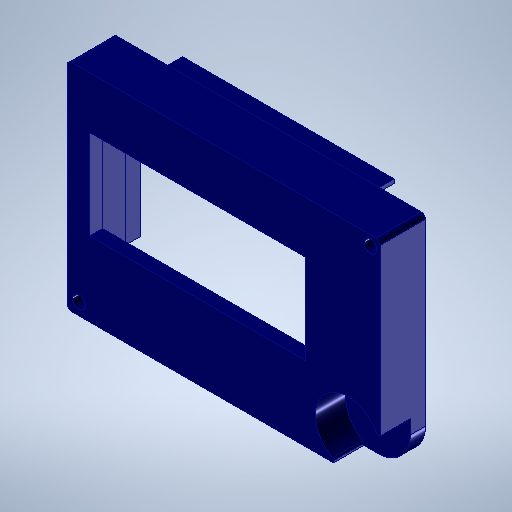
# Autodesk Inventor part: Krabička_horni
Saved by Autodesk Inventor 2025.2 (Build 292293000, 293)
## iProperties
Created: 2025-03-25
Part Number: Krabička_horni
Material: Všeobecné
Document SubType Name: Modeling
Designer: jakub
Density: 1 g/cm^3
Appearance: Modrá – nástěnná malba – lesklá
Author: jakub
## iProperties of the stored document Krabička_horni_3D tisk.ipt
Created: 2025-03-26
Part Number: Krabička_horni_3D tisk
Material: Všeobecné
Document SubType Name: Modeling
Designer: jakub
Density: 1 g/cm^3
Appearance: Výchozí
Author: jakub
Autodesk Inventor part; units mm, degrees
ref_plane "YZ Plane" through (0, 0, 0) normal (1, 0, 0) x (0, 1, 0)
ref_plane "XZ Plane" through (0, 0, 0) normal (0, 1, 0) x (-1, 0, 0)
ref_plane "XY Plane" through (0, 0, 0) normal (0, 0, 1) x (1, 0, 0)
sketch "Náčrt1" plane through (0, 0, 0) normal (0, 0, 1) x (1, 0, 0)
  line L0 (0, 71.1184) -> (0, -73.8108) projected
  line L1 (-102.6184, 0) -> (105.3108, 0) projected
  line L2 (-72.5, 50) -> (72.5, 50)
  line L3 (72.5, 50) -> (72.5, -35)
  line L4 (57.5, -50) -> (-72.5, -50)
  line L5 (-72.5, -50) -> (-72.5, 50)
  arc A0 (57.5, -50) -> (72.5, -35) centre (57.5, -35) ccw
  point P0 (0, 0)
  dimension "d2" = 30
  dimension "d37" = 145
  dimension "d38" = 100
  constraints: 8 end point, 2 parallel, 2 point on circle, 2 tangent, 1 centre point, 1 horizontal, 1 perpendicular, 2 other
  measures "d2" diameter of A0
  measures "d37" distance between parallel lines of L3 L5
  measures "d38" distance between parallel lines of L2 L4
extrude "Vysunutí1" add sketch "Náčrt1" along normal blind 21
sketch "Náčrt2" plane through (0, 0, 21) normal (0, 0, 1) x (1, 0, 0)
  line L0 (-72.5, -50) -> (57.5, -50) projected
  arc A0 (57.5, -50) -> (72.5, -35) centre (57.5, -35) ccw projected
  line L1 (72.5, -35) -> (72.5, 50) projected
  line L2 (72.5, 50) -> (-72.5, 50) projected
  line L3 (-72.5, 50) -> (-72.5, -50) projected
  circle A1 centre (57.5, -35) radius 15
  line L4 (72.5, -27.3264) -> (72.5, -35)
  line L5 (64.2851, -50) -> (57.5, -50)
  line L6 (72.5, -35) -> (72.5, 50) projected
  line L7 (72.5, -35) -> (72.5, -35)
  line L8 (72.5, -28.4617) -> (71, -28.4617)
  line L9 (50.9617, -48.5) -> (50.9617, -50)
  point P0 (0, 0)
  point P1 (49.2851, -47.5505)
  point P2 (70.3886, -27.3264)
  point P3 (50.9617, -50)
  dimension "d11" = 1.5
  dimension "d12" = 1.5
  constraints: 10 end point, 5 point on circle, 5 point on line, 4 perpendicular, 4 tangent, 1 centre point, 1 coincident, 1 collinear, 1 concentric
  measures "d11" distance of L8.start L8.end
  measures "d12" distance of L9.start L9.end
extrude "Vysunutí2" cut sketch "Náčrt2" against normal blind 14 contours L9 A1 L0 | A1 A0 | A1 L8 L1
sketch "Náčrt3" plane through (0, 0, 7) normal (0, 0, 1) x (1, 0, 0)
  arc A0 (57.5, -50) -> (72.5, -35) centre (57.5, -35) ccw projected
  circle A1 centre (57.5, -35) radius 4.25
  line L0 (72.5, -28.4617) -> (72.5, -35) projected
  line L1 (57.5, -50) -> (50.9617, -50) projected
  line L2 (71, -28.4617) -> (72.5, -28.4617) projected
  arc A2 (71, -28.4617) -> (50.9617, -48.5) centre (57.5, -35) ccw projected
  line L3 (50.9617, -50) -> (50.9617, -48.5) projected
  point P0 (0, 0)
  dimension "d7" = 8.5
  constraints: 1 centre point, 1 coincident
  measures "d7" diameter of A1
extrude "Vysunutí3" cut sketch "Náčrt3" against normal blind 12 contours A1
fillet "Zaoblení1" radius 2 3 edges at (72.5, 50, 10.5) (-72.5, 50, 10.5) (-72.5, -50, 10.5)
fillet "Zaoblení2" radius 1 2 edges at (71, -28.4617, 14) (50.9617, -48.5, 14)
sketch "Náčrt4" plane through (0, 0, 21) normal (0, 0, 1) x (1, 0, 0)
  arc A0 (50.9617, -49.1129) -> (50.4328, -48.2308) centre (49.9617, -49.1129) ccw projected
  arc A1 (70.7308, -27.9328) -> (50.4328, -48.2308) centre (57.5, -35) ccw projected
  arc A2 (70.7308, -27.9328) -> (71.6129, -28.4617) centre (71.6129, -27.4617) ccw projected
  line L0 (71.6129, -28.4617) -> (72.5, -28.4617) projected
  line L1 (72.5, -28.4617) -> (72.5, 48) projected
  arc A3 (72.5, 48) -> (70.5, 50) centre (70.5, 48) ccw projected
  line L2 (70.5, 50) -> (-70.5, 50) projected
  arc A4 (-70.5, 50) -> (-72.5, 48) centre (-70.5, 48) ccw projected
  line L3 (-72.5, 48) -> (-72.5, -48) projected
  arc A5 (-72.5, -48) -> (-70.5, -50) centre (-70.5, -48) ccw projected
  line L4 (-70.5, -50) -> (50.9617, -50) projected
  line L5 (50.9617, -50) -> (50.9617, -49.1129) projected
  line L6 (-66.5, 44) -> (68.5, 44) construction
  line L7 (68.5, 44) -> (68.5, -44) construction
  line L8 (68.5, -44) -> (-66.5, -44) construction
  line L9 (-66.5, -44) -> (-66.5, 44) construction
  point P0 (0, 0)
  dimension "d14" = 4
  dimension "d15" = 6
  dimension "d16" = 6
  dimension "d17" = 6
  constraints: 8 end point, 2 parallel, 1 horizontal, 1 perpendicular
  measures "d14" distance between parallel lines of L1 L7
  measures "d15" distance between parallel lines of L4 L8
  measures "d16" distance between parallel lines of L6 L2
  measures "d17" distance between parallel lines of L3 L9
sketch "Náčrt5" plane through (0, 0, 21) normal (0, 0, 1) x (1, 0, 0)
  line L0 (-62.1, 26) -> (37.9, 26)
  line L1 (37.9, 26) -> (37.9, -15.5)
  line L2 (37.9, -15.5) -> (-62.1, -15.5)
  line L3 (-62.1, -15.5) -> (-62.1, 26)
  line L4 (-66.5, 44) -> (68.5, 44) construction
  line L5 (-66.5, -44) -> (-66.5, 44) construction
  line L6 (68.5, -44) -> (-66.5, -44) construction
  line L7 (68.5, 44) -> (68.5, -44) construction
  point P0 (0, 0)
  dimension "d18" = 100
  dimension "d19" = 41.5
  dimension "d20" = 18
  dimension "d21" = 4.4
  constraints: 8 end point, 2 parallel, 1 horizontal, 1 perpendicular
  measures "d18" distance of L1.end L2.end
  measures "d19" distance between parallel lines of L2 L0
  measures "d20" distance between parallel lines of L0 L4
  measures "d21" distance between parallel lines of L5 L3
extrude "Vysunutí4" cut sketch "Náčrt5" against normal blind 21
sketch "Náčrt6" plane through (0, 0, 0) normal (0, 0, -1) x (-1, 0, 0)
  line L0 (-37.9, -15.5) -> (-37.9, 26) projected
  line L1 (-37.9, 26) -> (62.1, 26) projected
  line L2 (62.1, 26) -> (62.1, -15.5) projected
  line L3 (62.1, -15.5) -> (-37.9, -15.5) projected
  arc A0 (70.5, -50) -> (72.5, -48) centre (70.5, -48) ccw projected
  line L4 (72.5, 48) -> (72.5, -48) projected
  arc A1 (72.5, 48) -> (70.5, 50) centre (70.5, 48) ccw projected
  line L5 (-70.5, 50) -> (70.5, 50) projected
  arc A2 (-70.5, 50) -> (-72.5, 48) centre (-70.5, 48) ccw projected
  line L6 (-72.5, -35) -> (-72.5, 48) projected
  arc A3 (-72.5, -35) -> (-57.5, -50) centre (-57.5, -35) ccw projected
  line L7 (70.5, -50) -> (-57.5, -50) projected
  circle A4 centre (-57.5, -35) radius 4.25 projected
  arc A5 (-50.4328, -48.2308) -> (-70.7308, -27.9328) centre (-57.5, -35) ccw projected
  line L8 (0, -73.8108) -> (0, 71.1184) projected
  line L9 (-105.3108, 0) -> (102.6184, 0) projected
  line L10 (-68.5, 44) -> (66.5, 44)
  line L11 (66.5, 44) -> (66.5, -44)
  line L12 (66.5, -44) -> (-42.4917, -44)
  line L13 (-68.5, -24.802) -> (-68.5, 44)
  arc A6 (-42.4917, -44) -> (-68.5, -21.3893) centre (-57.5, -35) ccw
  point P0 (0, 0)
  dimension "d24" = 4
  dimension "d25" = 6
  dimension "d26" = 6
  dimension "d27" = 6
  dimension "d28" = 35
  constraints: 8 end point, 3 point on circle, 2 parallel, 1 centre point, 1 coincident, 1 horizontal, 1 perpendicular, 1 point on line
  measures "d24" distance between parallel lines of L6 L13
  measures "d25" distance between parallel lines of L10 L5
  measures "d26" distance between parallel lines of L11 L4
  measures "d27" distance between parallel lines of L7 L12
  measures "d28" diameter of A6
extrude "Vysunutí5" cut sketch "Náčrt6" against normal blind 17 contours L3 L8 L12 A6 L13 L9 L0 | L9 L13 L10 L8 L1 L0 | L3 L2 L9 L11 L12 L8 | L8 L10 L11 L9 L2 L1
sketch "Náčrt7" plane through (0, 0, 17) normal (0, 0, -1) x (-1, 0, 0)
  line L0 (-68.5, 44) -> (66.5, 44) projected
  line L1 (-68.5, -21.3893) -> (-68.5, 44) projected
  arc A0 (-42.4917, -44) -> (-68.5, -21.3893) centre (-57.5, -35) ccw projected
  line L2 (66.5, -44) -> (-42.4917, -44) projected
  line L3 (66.5, 44) -> (66.5, -44) projected
  line L4 (62.1, -15.5) -> (62.1, 26) projected
  line L5 (-37.9, -15.5) -> (62.1, -15.5) projected
  line L6 (-37.9, 26) -> (-37.9, -15.5) projected
  line L7 (62.1, 26) -> (-37.9, 26) projected
  line L8 (-40.4, 28.5) -> (64.6, 28.5)
  line L9 (64.6, 28.5) -> (64.6, -18)
  line L10 (64.6, -18) -> (-40.4, -18)
  line L11 (-40.4, -18) -> (-40.4, 28.5)
  point P0 (0, 0)
  dimension "d31" = 2.5
  dimension "d32" = 2.5
  dimension "d33" = 2.5
  dimension "d34" = 2.5
  constraints: 8 end point, 2 parallel, 1 horizontal, 1 perpendicular
  measures "d31" distance between parallel lines of L11 L6
  measures "d32" distance between parallel lines of L7 L8
  measures "d33" distance between parallel lines of L4 L9
  measures "d34" distance between parallel lines of L10 L5
extrude "Vysunutí6" add sketch "Náčrt7" along normal blind 2 contours L8 L9 L10 L11
sketch "Náčrt8" plane through (0, 0, 0) normal (0, 0, -1) x (-1, 0, 0)
  line L0 (-68.5, -21.3893) -> (-68.5, 44) projected
  line L1 (-68.5, 44) -> (66.5, 44) projected
  line L2 (66.5, 44) -> (66.5, -44) projected
  line L3 (66.5, -44) -> (-42.4917, -44) projected
  arc A0 (-42.4917, -44) -> (-68.5, -21.3893) centre (-57.5, -35) ccw projected
  arc A1 (70.5, -50) -> (72.5, -48) centre (70.5, -48) ccw projected
  line L4 (72.5, 48) -> (72.5, -48) projected
  arc A2 (72.5, 48) -> (70.5, 50) centre (70.5, 48) ccw projected
  line L5 (-70.5, 50) -> (70.5, 50) projected
  arc A3 (-70.5, 50) -> (-72.5, 48) centre (-70.5, 48) ccw projected
  line L6 (-72.5, -35) -> (-72.5, 48) projected
  arc A4 (-72.5, -35) -> (-57.5, -50) centre (-57.5, -35) ccw projected
  line L7 (70.5, -50) -> (-57.5, -50) projected
  circle A5 centre (-57.5, -35) radius 4.25 projected
  point P0 (0, 0)
sketch "Náčrt9" plane through (0, 0, 17) normal (0, 0, -1) x (-1, 0, 0)
  line L0 (-40.4, -18) -> (-40.4, 28.5) projected
  line L1 (-40.4, 28.5) -> (64.6, 28.5) projected
  line L2 (64.6, 28.5) -> (64.6, -18) projected
  line L3 (64.6, -18) -> (-40.4, -18) projected
  line L4 (-68.5, 44) -> (66.5, 44) projected
  line L5 (-68.5, -21.3893) -> (-68.5, 44) projected
  arc A0 (-42.4917, -44) -> (-68.5, -21.3893) centre (-57.5, -35) ccw projected
  line L6 (66.5, -44) -> (-42.4917, -44) projected
  line L7 (66.5, 44) -> (66.5, -44) projected
  line L8 (66.5, -44) -> (-42.4917, -44) projected
  line L9 (66.5, -44) -> (62, -44)
  line L10 (62, -44) -> (62, -40.5)
  line L11 (62, -40.5) -> (66.5, -40.5)
  line L12 (66.5, -40.5) -> (66.5, -44)
  line L13 (-68.5, 44) -> (-63, 44)
  line L14 (-63, 44) -> (-63, 38.5)
  line L15 (-63, 38.5) -> (-68.5, 38.5)
  line L16 (-68.5, 38.5) -> (-68.5, 44)
  point P0 (0, 0)
  dimension "d48" = 4.5
  dimension "d49" = 3.5
  dimension "d50" = 5.5
  dimension "d51" = 5.5
  constraints: 16 end point, 4 parallel, 2 horizontal, 2 perpendicular
  measures "d48" distance of L10.end L11.end
  measures "d49" distance of L9.end L10.end
  measures "d50" distance of L14.end L15.end
  measures "d51" distance of L13.end L14.end
extrude "Vysunutí7" add sketch "Náčrt9" along normal up to surface (17 mm away) contours L4 L14 L15 L5 | L7 L6 L10 L11
sketch "Náčrt10" plane through (0, 0, 0) normal (0, 0, -1) x (-1, 0, 0)
  circle A0 centre (67, -44.5) radius 3
  circle A1 centre (-68, 45.5) radius 3
  line L0 (-72.5, -35) -> (-72.5, 48) projected
  line L1 (-70.5, 50) -> (70.5, 50) projected
  line L2 (70.5, -50) -> (-57.5, -50) projected
  line L3 (72.5, 48) -> (72.5, -48) projected
  point P0 (0, 0)
  dimension "d54" = 6
  dimension "d55" = 6
  dimension "d56" = 4.5
  dimension "d57" = 4.5
  dimension "d58" = 5.5
  dimension "d59" = 5.5
  constraints: 2 centre point
  measures "d54" diameter of A0
  measures "d55" diameter of A1
  measures "d56" distance from line of L0 A1.centre
  measures "d57" distance from line of L1 A1.centre
  measures "d58" distance from line of L2 A0.centre
  measures "d59" distance from line of L3 A0.centre
sketch "Náčrt11" plane through (0, 0, 21) normal (0, 0, 1) x (1, 0, 0)
  point P0 (0, 0)
  point P1 (-67, -44.5)
  point P2 (68, 45.5)
  point P3 (68, 45.5)
  point P4 (-67, -44.5)
  constraints: 2 coincident
hole "Díra1" at (68, 45.5, 21) at (-67, -44.5, 21) direction (0, 0, -1) diameter 6 depth 17
sketch "Náčrt12" plane through (68, 45.5, 4) normal (0, 0, 1) x (1, 0, 0)
  line L0 (4.5, -73.9617) -> (4.5, 2.5) projected
  line L1 (2.5, 4.5) -> (-138.5, 4.5) projected
  circle A0 centre (-135, -90) radius 3 projected
  point P0 (-68, -45.5)
  point P1 (0, 0)
  dimension "d67" = 4.5
  dimension "d68" = 4.5
  constraints: 1 coincident
  measures "d67" distance from line of L0 point (0, 0)
  measures "d68" distance from line of L1 point (0, 0)
hole "Díra2" at (68, 45.5, 4) at (-67, -44.5, 4) direction (0, 0, -1) diameter 3.3 depth 17
sketch "Náčrt13" plane through (0, 0, 0) normal (0, 0, -1) x (-1, 0, 0)
  line L0 (49, -47.925) -> (-49, -47.925)
  line L1 (-49, -47.925) -> (-49, -46.075)
  line L2 (-49, -46.075) -> (49, -46.075)
  line L3 (49, -46.075) -> (49, -47.925)
  line L4 (0, -73.8108) -> (0, 71.1184) projected
  line L5 (70.5, -50) -> (-57.5, -50) projected
  line L6 (-105.3108, 0) -> (102.6184, 0) projected
  line L7 (49, 47.925) -> (-49, 47.925)
  line L8 (-49, 47.925) -> (-49, 46.075)
  line L9 (-49, 46.075) -> (49, 46.075)
  line L10 (49, 46.075) -> (49, 47.925)
  line L11 (70.425, -34) -> (68.575, -34)
  line L12 (68.575, -34) -> (68.575, 34)
  line L13 (68.575, 34) -> (70.425, 34)
  line L14 (70.425, 34) -> (70.425, -34)
  line L15 (66.5, 44) -> (66.5, -40.5) projected
  point P0 (0, 0)
  dimension "d76" = 98
  dimension "d77" = 1.85
  dimension "d78" = 2.075
  dimension "d79" = 1.85
  dimension "d80" = 68
  dimension "d81" = 2.075
  constraints: 24 end point, 4 parallel, 4 symmetric about line, 2 horizontal, 2 perpendicular, 2 other
  measures "d76" distance of L1.end L2.end
  measures "d77" distance between parallel lines of L2 L0
  measures "d78" distance between parallel lines of L5 L0
  measures "d79" distance of L12.end L13.end
  measures "d80" distance of L11.end L12.end
  measures "d81" distance between parallel lines of L15 L12
extrude "Vysunutí8" add sketch "Náčrt13" along normal blind 9
